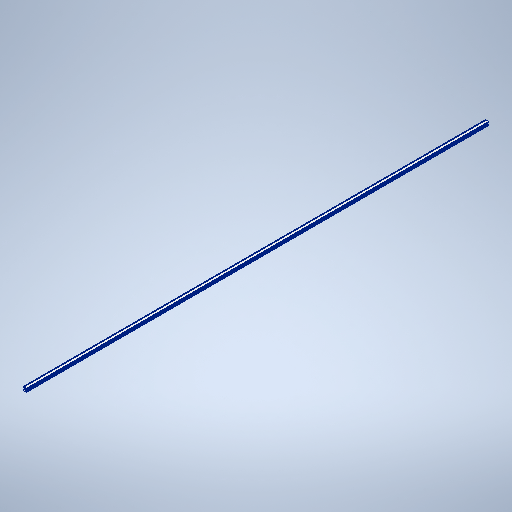
# Autodesk Inventor part: 15×15 2 slots profile_AST01501502
Saved by Autodesk Inventor 2025.2 (Build 292293000, 293)
## iProperties
Created: 2025-03-25
Part Number: 15×15 2 slots profile_AST01501502
Material: Polietileno, Alta Densidade
Document SubType Name: Modeling
Designer: lucas
Density: 0.952 g/cm^3
Appearance: Alumínio - Plano
Author: lucas
Autodesk Inventor part; units mm, degrees
ref_plane "YZ Plane" through (0, 0, 0) normal (1, 0, 0) x (0, 1, 0)
ref_plane "XZ Plane" through (0, 0, 0) normal (0, 1, 0) x (-1, 0, 0)
ref_plane "XY Plane" through (0, 0, 0) normal (0, 0, 1) x (1, 0, 0)
sketch "Esboço1" plane through (0, 0, 0) normal (0, 0, 1) x (1, 0, 0)
  line L0 (7.5, 7.5) -> (-7.5, 7.5) construction
  line L1 (-7.5, 3.1) -> (-7.5, -3.1) construction
  line L2 (-7.5, 7.5) -> (-7.5, 3.1) construction
  line L3 (-7.5, 3.1) -> (-5.5, 3.1) construction
  line L4 (-5.5, 3.1) -> (-5.5, 6.2) construction
  line L5 (-5.5, 6.2) -> (-1.5, 3.1) construction
  line L6 (-1.5, 3.1) -> (-1.5, 0) construction
  line L7 (-1.5, 0) -> (0, 0)
  line L8 (0, 0) -> (0, 7.5)
  arc A0 (-7, 7.5) -> (-7.5, 7) centre (-7, 7) ccw
  line L9 (-7.5, 3.1) -> (-7, 3.1) construction
  line L10 (-7, 3.1) -> (-7, 3.6)
  line L11 (-7, 3.6) -> (-7.5, 3.6)
  line L12 (-7.5, 3.6) -> (-7.5, 3.1) construction
  line L13 (-7.5, 7) -> (-7.5, 3.6)
  line L14 (-7, 7.5) -> (0, 7.5)
  line L15 (-7, 3.1) -> (-5.5, 3.1)
  arc A1 (-5.1775, 5.9501) -> (-5.5, 5.792) centre (-5.3, 5.792) ccw
  line L16 (-5.5, 3.1) -> (-5.5, 5.792)
  arc A2 (-1.5, 2.8549) -> (-1.6937, 3.2501) centre (-2, 2.8549) ccw
  line L17 (-5.1775, 5.9501) -> (-1.6937, 3.2501)
  line L18 (-1.5, 2.8549) -> (-1.5, 0)
  point P0 (-7.5, 0)
  dimension "d0" = 15
  dimension "d1" = 6.2
  dimension "d2" = 7.5
  dimension "d4" = 2
  dimension "d5" = 6
  dimension "d7" = 3.1
  dimension "d10" = 0.5
  dimension "d11" = 0.5
  dimension "d12" = 0.2
  dimension "d13" = 0.5
  constraints: 38 end point, 7 tangent, 6 collinear, 6 point on circle, 6 point on line, 4 perpendicular, 4 vertical, 3 centre point, 3 horizontal, 2 horizontal alignment, 2 midpoint, 2 parallel, 1 vertical alignment
  measures "d0" distance of L0.start L0.end
  measures "d1" distance of L1.start L1.end
  measures "d2" distance from line of L7.end L0
  measures "d4" distance of L1.start L3.end
  measures "d5" distance of L1.start L5.end
  measures "d7" distance of L3.end L4.end
  measures "d10" radius of A0
  measures "d11" distance of L10.end L11.end
  measures "d12" radius of A1
  measures "d13" radius of A2
extrude "Extrusão1" add sketch "Esboço1" along normal mid plane 2000
mirror "Espelhar1" about plane through (0, 0, 0) normal (1, 0, 0) of "Extrusão1"
mirror "Espelhar2" about plane through (0, 0, 0) normal (0, 1, 0) of "Extrusão1", "Espelhar1"
equation "\"d2\" = 0.5 * d0"
